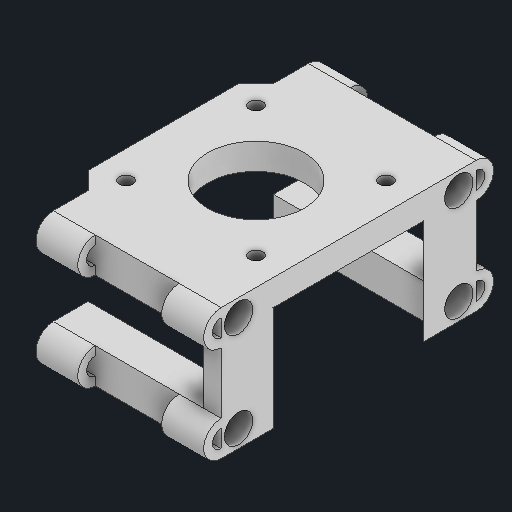
# Autodesk Inventor part: carriage_motor_mount
Saved by Autodesk Inventor 2025 (Build 290162010, 162A)
## iProperties
Created: 2024-07-11
Part Number: carriage_motor_mount
Material: Generic
Document SubType Name: Modeling
Designer: mihir
Density: 1 g/cm^3
Appearance: Default
Author: mihir
Autodesk Inventor part; units mm, degrees
ref_plane "YZ Plane" through (0, 0, 0) normal (1, 0, 0) x (0, 1, 0)
ref_plane "XZ Plane" through (0, 0, 0) normal (0, 1, 0) x (-1, 0, 0)
ref_plane "XY Plane" through (0, 0, 0) normal (0, 0, 1) x (1, 0, 0)
sketch "Sketch1" plane through (0, 0, 0) normal (0, 1, 0) x (-1, 0, 0)
  circle A0 centre (0, 0) radius 11.05
  line L0 (17.25, 21.25) -> (21.25, 17.25)
  line L1 (21.25, 17.25) -> (21.25, -17.25)
  line L2 (21.25, -17.25) -> (17.25, -21.25)
  line L3 (17.25, -21.25) -> (-17.25, -21.25)
  line L4 (-17.25, -21.25) -> (-21.25, -17.25)
  line L5 (-21.25, -17.25) -> (-21.25, 17.25)
  line L6 (-21.25, 17.25) -> (-17.25, 21.25)
  line L7 (-17.25, 21.25) -> (17.25, 21.25)
  line L8 (0, 21.25) -> (0, -21.25) construction
  line L9 (21.25, 0) -> (-21.25, 0) construction
  circle A1 centre (14.8987, 14.8987) radius 1.55
  line L10 (14.8987, 14.8987) -> (0, 0) construction
  circle A2 centre (-14.8987, 14.8987) radius 1.55
  circle A3 centre (-14.8987, -14.8987) radius 1.55
  circle A4 centre (14.8987, -14.8987) radius 1.55
  dimension "d0" = 22.1
  dimension "d1" = 42.5
  dimension "d2" = 4
  dimension "d3" = 135
  dimension "d4" = 3.1
  dimension "d5" = 21.07
  dimension "d6" = 45
  dimension "d9" = 360
  constraints: 22 end point, 7 perpendicular, 6 midpoint, 5 centre point, 2 coincident, 2 horizontal, 2 vertical, 9 other
  measures "d0" diameter of A0
  measures "d1" distance between parallel lines of L3 L7
  measures "d2" horizontal distance of L0.start L0.end
  measures "d4" diameter of A1
  measures "d5" distance of L10.start L10.end
extrude "Extrusion1" add sketch "Sketch1" along normal blind 6
sketch "Sketch2" plane through (0, 6, 0) normal (0, 1, 0) x (1, 0, 0)
  line L0 (-21.25, -17.25) -> (-17.25, -21.25) projected
  line L1 (-17.25, -21.25) -> (-17.25, -29.25)
  line L2 (-17.25, -29.25) -> (21.25, -29.25)
  line L3 (21.25, -29.25) -> (21.25, 29.25)
  line L4 (21.25, 29.25) -> (-17.25, 29.25)
  line L5 (17.25, 21.25) -> (-17.25, 21.25) projected
  line L6 (-17.25, 29.25) -> (-17.25, 21.25)
  line L7 (-17.25, 21.25) -> (17.25, 21.25)
  line L8 (21.25, 17.25) -> (17.25, 21.25) projected
  line L9 (17.25, 21.25) -> (21.25, 17.25)
  line L10 (21.25, 17.25) -> (21.25, -17.25)
  line L11 (21.25, -17.25) -> (17.25, -21.25)
  line L12 (17.25, -21.25) -> (-17.25, -21.25)
  line L13 (21.25, -17.25) -> (21.25, 17.25) projected
  point P0 (0, 0)
  point P1 (21.25, -17.25)
  dimension "d13" = 8
  constraints: 20 end point, 6 perpendicular, 4 collinear, 1 parallel, 1 point on line, 1 vertical
  measures "d13" distance of L0.end L1.end
extrude "Extrusion2" add sketch "Sketch2" against normal blind 8
sketch "Sketch3" plane through (0, -2, 0) normal (0, -1, 0) x (1, 0, 0)
  line L0 (21.25, 29.25) -> (21.25, -29.25) projected
  line L1 (21.25, -17.25) -> (17.25, -21.25) projected
  line L2 (21.25, -29.25) -> (21.25, -17.25)
  line L3 (21.25, -17.25) -> (17.25, -21.25)
  line L4 (17.25, -21.25) -> (17.25, -29.25)
  line L5 (17.25, -29.25) -> (21.25, -29.25)
  line L6 (17.25, 21.25) -> (21.25, 17.25) projected
  line L7 (21.25, 17.25) -> (17.25, 21.25)
  line L8 (17.25, 21.25) -> (17.25, 29.25)
  line L9 (21.25, 29.25) -> (-17.25, 29.25) projected
  line L10 (21.25, 29.25) -> (21.25, 17.25)
  point P0 (0, 0)
  constraints: 14 end point, 3 collinear, 2 vertical, 1 parallel, 1 perpendicular, 1 point on line
extrude "Extrusion3" add sketch "Sketch3" along normal blind 22
sketch "Sketch4" plane through (17.25, -2, 21.25) normal (-1, 0, 0) x (0, 0, 1)
  line L0 (8, 8) -> (8, -22) projected
  line L1 (0, 0) -> (0, -22) projected
  line L2 (8, -22) -> (0, -22)
  line L3 (0, -22) -> (0, -14)
  line L4 (0, -14) -> (8, -14)
  line L5 (8, -14) -> (8, -22)
  line L6 (-42.5, 0) -> (-42.5, -22) projected
  line L7 (-50.5, 8) -> (-50.5, -22) projected
  line L8 (-42.5, -22) -> (-50.5, -22)
  line L9 (-50.5, -22) -> (-50.5, -14)
  line L10 (-50.5, -14) -> (-42.5, -14)
  line L11 (-42.5, -14) -> (-42.5, -22)
  point P0 (-21.25, 2)
  point P1 (8, -14)
  dimension "d18" = 8
  constraints: 16 end point, 4 parallel, 2 horizontal, 2 perpendicular, 2 point on line, 1 collinear
  measures "d18" distance between parallel lines of L4 L2
extrude "Extrusion4" add sketch "Sketch4" along normal up to surface (34.5 mm away)
sketch "Sketch5" plane through (-17.25, -24, -21.25) normal (-1, 0, 0) x (0, 0, 1)
  line L0 (-8, 8) -> (0, 8) construction
  line L1 (-4, 8) -> (-4, 0) construction
  line L2 (-8, 0) -> (4, 0) construction
  circle A0 centre (-4, 4) radius 3.25
  line L3 (-8, 0) -> (-8, 8) construction
  line L4 (-8, 4) -> (-4, 4) construction
  circle A1 centre (-4, 26) radius 3.25
  circle A2 centre (46.5, 4) radius 3.25
  circle A3 centre (46.5, 26) radius 3.25
  point P0 (21.25, 24)
  dimension "d21" = 6.5
  dimension "d24" = 22
  dimension "d27" = 50.5
  constraints: 4 centre point, 4 end point, 3 midpoint, 2 vertical, 1 horizontal, 1 perpendicular, 1 point on line, 6 other
  measures "d21" diameter of A0
  measures "d24" distance of L4.end A1.centre
  measures "d27" distance of L4.end A2.centre
extrude "Extrusion5" cut sketch "Sketch5" against normal up to surface (38.5 mm away)
sketch "Sketch6" plane through (-17.25, -24, 29.25) normal (-1, 0, 0) x (0, 0, 1)
  arc A0 (0, 2) -> (0, 6) centre (0, 4) ccw
  arc A1 (0, 0) -> (0, 8) centre (0, 4) ccw
  line L0 (0, 0) -> (0, 2)
  line L1 (0, 6) -> (0, 8)
  line L2 (0, 8) -> (0, 0) projected
  point P0 (-29.25, 24)
  dimension "d32" = 2
  dimension "d34" = 180
  constraints: 4 end point, 4 point on circle, 2 centre point, 2 collinear, 1 concentric, 1 vertical
  measures "d32" radial gap between concentric circles of A1 A0
extrude "Extrusion6" add sketch "Sketch6" against normal up to surface (38.5 mm away) contours A0 L1 A1 L0
ref_plane "Work Plane1" through (0, -9, 0) normal (0, -1, 0) x (1, 0, 0)
ref_plane "Work Plane2" through (-17.25, 6, 0) normal (0, 0, 1) x (1, 0, 0)
ref_plane "Work Plane3" through (2, 6, 29.25) normal (1, 0, 0) x (0, 0, -1)
mirror "Mirror1" about plane through (0, -9, 0) normal (0, -1, 0) of "Extrusion6"
mirror "Mirror2" about plane through (-17.25, 6, 0) normal (0, 0, 1) of "Extrusion6", "Mirror1"
sketch "Sketch7" plane through (2, 6, 29.25) normal (1, 0, 0) x (0, 0, -1)
  line L0 (12, -30) -> (0, -30) projected
  line L1 (0, -30) -> (-4, -30)
  line L2 (-4, -30) -> (-4, 0)
  line L3 (-4, 0) -> (0, 0)
  line L4 (0, 0) -> (0, -30)
  arc A0 (0, -22) -> (0, -30) centre (0, -26) ccw projected
  arc A1 (58.5, -30) -> (58.5, -22) centre (58.5, -26) ccw projected
  line L5 (58.5, -30) -> (62.5, -30)
  line L6 (62.5, -30) -> (62.5, 0)
  line L7 (62.5, 0) -> (58.5, 0)
  line L8 (58.5, 0) -> (58.5, -30)
  point P0 (29.25, -6)
  constraints: 16 end point, 4 parallel, 2 horizontal, 2 perpendicular, 2 tangent
extrude "Extrusion7" cut sketch "Sketch7" along normal mid plane 19.25
equation "\"d11\" = mount_face_thickness"
equation "\"d13\" = post_width"
equation "\"d14\" = post_width"
equation "\"d16\" = mount_length - post_width"
equation "\"d18\" = post_width"
equation "\"d19\" = mount_length - post_width"
equation "\"d21\" = rod_diameter + rod_free_tolerance"
equation "\"d24\" = mount_length - post_width"
equation "\"mount_face_thickness\" = 6"
equation "\"post_width\" = 8"
equation "\"slider_rod_diameter\" = 5"
equation "\"rod_diameter\" = 6"
equation "\"rod_free_tolerance\" = 0.5"
equation "\"mount_length\" = 30"
body "Solid1"
